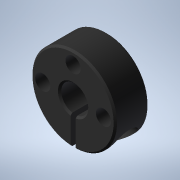
# Autodesk Inventor part: SCST8-10b
Saved by Autodesk Inventor 2021 (Build 250183000, 183)
## iProperties
Created: 2025-08-06
Part Number: SCST8-10b
Material: Generic
Catalog Web Link: www.cadenas.de
Description: SCST, PSCST, SSCST, SCSTR, PSCSTR, SSCSTR-b-Set Collars - Slit 3 Hole/3 Tap - Standard Type -
Vendor: MISUMI
Document SubType Name: Modeling
Designer: psAdmin
Manufacturer: MISUMI
Mass: 3.44673 g
Surface Area: 24.7262 cm^2
Volume: 3.44673 cm^3
Density: 1 g/cm^3
Appearance: PSOLRGB-175-175-175
Category: PARTsolutions
Company: MISUMI
Title: SCST8-10
Author: Cadenas PARTsolutions
Comments: Set Collars - Slit 3 Hole/3 Tap - Standard Type -
PSOL_IDENT_0: {$CADENAS_DATA/23d-libs/misumi/metric/03_set_collars/scst/scst_b.prj},208 {VTYP=3D},{NB=SCST8-10b},{
PSOL_IDENT_1: LINA=SCST8-10},{NN=SCST, PSCST, SSCST, SCSTR, PSCSTR, SSCSTR-b},{DATE=29.11.2024 04:05:20},{GEOMDATE=
PSOL_IDENT_2: 15.09.2021 06:06:07},{VERSION=},{LINEID=50},{WBVAR=TS,MAT,ST,BS},{WBNUMERIC=BS}  {NB=SCST8-10b},{LIN
PSOL_IDENT_3: A=SCST8-10},{KT=DUMMY},{PN=SCST8-10},{TYPE=SCST},{TS=3H},{TSALG= '3H' , '3-Hole' , '3T' , '3-Tapped'
PSOL_IDENT_4: },{TSA='3H', '3-Hole', '3T', '3 Tap (Coarse)'},{MAT=S45C},{ST=BO},{STALG= 'BO' , 'Black Oxide' , 'E
PSOL_IDENT_5: NP' , 'Electroless Nickel Plating' },{AC=Hex Socket Head Cap Screw 1 pc.},{ACMAT=4137 Alloy Steel},{
PSOL_IDENT_6: D=8},{BS=10},{BALG= 8 , 10 , 15 },{D1=25},{M=M4},{M3D=4},{DD=4.5},{R=3.75},{W=1.5},{X=8.0},{Y=5},{P=
PSOL_IDENT_7: 18},{C=0.5},{S=4.5},{M1=-},{M13D=0},{L=12}
NB: SCST8-10b
NN: SCST, PSCST, SSCST, SCSTR, PSCSTR, SSCSTR-b
NT: Set Collars - Slit 3 Hole/3 Tap - Standard Type -
NBSYN: $PN.b
LINA: SCST8-10
CATALOG: Misumi
PN: SCST8-10
TS: 3-Hole
MAT: 1045 Carbon Steel
ST: Black Oxide
AC: Hex Socket Head Cap Screw 1 pc.
ACMAT: 4137 Alloy Steel
D: 8
BS: 10
D1: 25
M: M4
DD: 4.5
R: 3.75
W: 1.5
X: 8
Y: 5
P: 18
C: 0.5
S: 4.5
M1: -
SUPPLIER: MISUMI
ARTICLENO: SCST8-10b
BOMINFO: SCST8-10
CREATOR: CADENAS GmbH
Autodesk Inventor part; units mm, degrees
sketch "Sketch_14" plane through (0, 0, 0) normal (1, 0, 0) x (0, 1, 0)
  line L0 (0, -5) -> (0, 5)
  line L1 (0, 5) -> (12, 5)
  line L2 (12, 5) -> (12.5, 4.5)
  line L3 (12.5, 4.5) -> (12.5, -4.5)
  line L4 (12.5, -4.5) -> (12, -5)
  line L5 (12, -5) -> (0, -5)
  line L6 (0, -5) -> (0, 5)
  constraints: 14 end point
revolve "Revolution1" add sketch "Sketch_14" angle 360 about axis through (0, 0, -5) along (0, 0, -1)
sketch "Sketch_15" plane through (0, 0, 0) normal (1, 0, 0) x (0, 1, 0)
  line L0 (0, -5) -> (0, 5)
  line L1 (0, 5) -> (4.5, 5)
  line L2 (4.5, 5) -> (4, 4.5)
  line L3 (4, 4.5) -> (4, -4.5)
  line L4 (4, -4.5) -> (4.5, -5)
  line L5 (4.5, -5) -> (0, -5)
  line L6 (0, -5) -> (0, 5)
  constraints: 14 end point
revolve "Revolution2" cut sketch "Sketch_15" angle 360 about axis through (0, 0, -5) along (0, 0, -1)
sketch "Sketch_16" plane through (0, 0, 0) normal (0, 0, 1) x (1, 0, 0)
  arc A0 (-0.75, -13.4792) -> (0.75, -13.4792) centre (0, 0) ccw
  line L0 (0.75, -13.4792) -> (0.75, 0)
  line L1 (0.75, 0) -> (-0.75, 0)
  line L2 (-0.75, 0) -> (-0.75, -13.4792)
  constraints: 6 end point, 2 point on circle, 1 centre point
extrude "Extrusion1" cut sketch "Sketch_16" along normal mid plane 10
sketch "Sketch4" plane through (0, 0, -5) normal (0, 0, -1) x (-1, 0, 0)
  point P0 (-9, 0)
hole "Hole1" at (9, 0, -5) direction (0, 0, 1) diameter 4.5 depth 10
sketch "Sketch5" plane through (0, 0, -5) normal (0, 0, -1) x (-1, 0, 0)
  point P0 (9, 0)
hole "Hole2" at (-9, 0, -5) direction (0, 0, 1) diameter 4.5 depth 10
sketch "Sketch6" plane through (0, 0, -5) normal (0, 0, -1) x (-1, 0, 0)
  point P0 (0, 9)
hole "Hole3" at (0, 9, -5) direction (0, 0, 1) diameter 4.5 depth 10
sketch "Sketch_23" plane through (0, -8, 0) normal (0, 1, 0) x (1, 0, 0)
  line L0 (12.5, 0) -> (0, 0)
  line L1 (0, 0) -> (0, 2.25)
  line L2 (0, 2.25) -> (5, 2.25)
  line L3 (5, 2.25) -> (5, 3.75)
  line L4 (5, 3.75) -> (12.5, 3.75)
  line L5 (12.5, 3.75) -> (12.5, 0)
  line L6 (12.5, 0) -> (0, 0)
  constraints: 14 end point
revolve "Revolution3" cut sketch "Sketch_23" angle 360 about axis through (12.5, -8, 0) along (1, 0, 0)
sketch "Sketch8" plane through (-0.75, -11.9765, 5) normal (1, 0, 0) x (0, 0, -1)
  point P0 (5, 3.9765)
hole "Hole4" at (-0.75, -8, 0) direction (-1, 0, 0) diameter 3.242 depth 10.2159 countersink diameter 4 countersink angle 90 thread size "M4x0.7" class "6H" standard "ISO Metric profile"
ref_plane "to_bolt_XY" through (5, -8, 0) normal (1, 0, 0) x (0, 0, -1)
ref_plane "to_bolt_YZ" through (5, -8, 0) normal (0, 0, -1) x (0, 1, 0)
ref_plane "to_bolt_ZX" through (5, -8, 0) normal (0, 1, 0) x (1, 0, 0)
body "Solid1"
